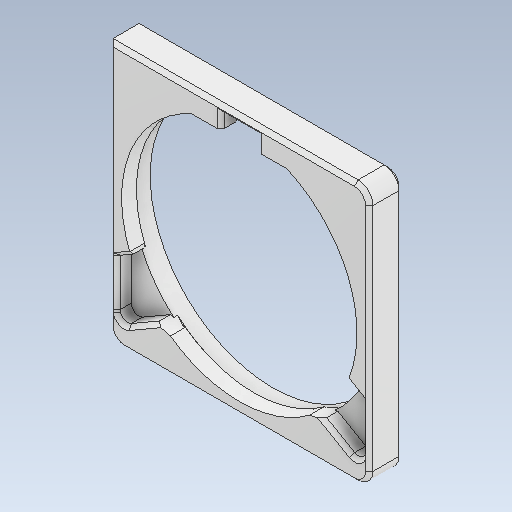
# Autodesk Inventor part: DD3_Zentrierhilfe
Saved by Autodesk Inventor 2020.2 (Build 242310000, 310)
## iProperties
Created: 2021-09-17
Part Number: DD3_Zentrierhilfe
Material: PC/ABS-Kunststoff
Document SubType Name: Modeling
Designer: johan
Density: 0.357273 g/cm^3
Appearance: Glatt - Weiß
Author: johan
Autodesk Inventor part; units mm, degrees
ref_plane "YZ Plane" through (0, 0, 0) normal (1, 0, 0) x (0, 1, 0)
ref_plane "XZ Plane" through (0, 0, 0) normal (0, 1, 0) x (-1, 0, 0)
sketch "Skizze1" plane through (0, 0, 0) normal (0, 0, 1) x (1, 0, 0)
  line L0 (-17, 17) -> (15.5, 17) construction
  line L1 (-17, -15.5) -> (-17, 17) construction
  arc A0 (-17, -15.5) -> (-15.5, -17) centre (-15.5, -15.5) ccw construction
  line L2 (15.5, -17) -> (-15.5, -17) construction
  arc A1 (15.5, -17) -> (17, -15.5) centre (15.5, -15.5) ccw construction
  line L3 (17, 15.5) -> (17, -15.5) construction
  arc A2 (17, 15.5) -> (15.5, 17) centre (15.5, 15.5) ccw construction
  arc A3 (-6.48479, 14.9) -> (6.48479, 14.9) centre (0, 0) ccw
  line L4 (6.48479, 14.9) -> (-6.48479, 14.9)
  line L5 (-2.5, 16.9) -> (2.5, 16.9)
  line L6 (2.5, 16.9) -> (2.5, 14.9)
  line L7 (2.5, 14.9) -> (-2.5, 14.9)
  line L8 (-2.5, 14.9) -> (-2.5, 16.9)
  line L9 (0, 0) -> (0, 20.018159) construction
  line L10 (0, 0) -> (0, -16.25) construction
  line L11 (0, 0) -> (-16.25, 0) construction
  line L12 (0, 0) -> (16.25, 0) construction
  line L13 (-16.5, -7.283583) -> (-13, -13.345761)
  line L14 (-13, -13.345761) -> (-11.267949, -12.345761)
  line L15 (-11.267949, -12.345761) -> (-14.767949, -6.283583)
  line L16 (-14.767949, -6.283583) -> (-16.5, -7.283583)
  line L17 (16.5, -7.283583) -> (13, -13.345761)
  line L18 (13, -13.345761) -> (11.267949, -12.345761)
  line L19 (11.267949, -12.345761) -> (14.767949, -6.283583)
  line L20 (14.767949, -6.283583) -> (16.5, -7.283583)
  line L21 (15.5, 17.5) -> (-17.5, 17.5)
  arc A4 (17.5, 15.5) -> (15.5, 17.5) centre (15.5, 15.5) ccw
  line L22 (17.5, -15.5) -> (17.5, 15.5)
  arc A5 (15.5, -17.5) -> (17.5, -15.5) centre (15.5, -15.5) ccw
  line L23 (-15.5, -17.5) -> (15.5, -17.5)
  arc A6 (-17.5, -15.5) -> (-15.5, -17.5) centre (-15.5, -15.5) ccw
  line L24 (-17.5, 17.5) -> (-17.5, -15.5)
  arc A7 (-6.400976, 14.5) -> (6.400976, 14.5) centre (0, 0) ccw
  line L25 (-6.400976, 14.5) -> (6.400976, 14.5)
  line L26 (-2.5, 14.9) -> (-2.5, 14.5)
  line L27 (2.5, 14.9) -> (2.5, 14.5)
  line L28 (14.767949, -6.283583) -> (14.767949, -5.755882)
  line L29 (11.267949, -12.345761) -> (9.430948, -12.738906)
  line L30 (-11.267949, -12.345761) -> (-9.284876, -12.845761)
  line L31 (-14.767949, -6.283583) -> (-14.767949, -5.755882)
  line L32 (13, -13.345761) -> (15.047939, -14.528139)
  line L33 (16.547911, -13.654594) -> (16.5, -7.283583)
  arc A8 (15.047939, -14.528139) -> (16.547911, -13.654594) centre (15.547939, -13.662114) ccw
  line L34 (-13, -13.345761) -> (-15.047939, -14.528139)
  line L35 (-16.547911, -13.654594) -> (-16.5, -7.283583)
  arc A9 (-16.547911, -13.654594) -> (-15.047939, -14.528139) centre (-15.547939, -13.662114) ccw
  point P0 (0, 0)
  point P1 (14.943148, -6.384734)
  point P2 (12.195347, -10.73946)
  point P3 (-12.195347, -10.73946)
  point P4 (-14.943148, -6.384734)
  dimension "d0" = 5
  dimension "d1" = 2
  dimension "d2" = 7
  dimension "d4" = 2
  dimension "d5" = 60
  dimension "d6" = 16.5
  dimension "d8" = 14.9
  dimension "d16" = 0.4
  dimension "d17" = 102.08
  dimension "d18" = 75.8487
  dimension "d19" = 20.23116
  dimension "d20" = 2.55685
  dimension "d21" = 23.88473
  dimension "d22" = 5.30465
  dimension "d23" = 28.23946
  dimension "d24" = 15
  dimension "d25" = 2.6
  dimension "d26" = 2.51816
  dimension "d27" = 20
  dimension "d28" = 2.6
  dimension "d29" = 29.69535
  dimension "d30" = 28.23946
  dimension "d31" = 32.44315
  dimension "d32" = 23.88473
  dimension "d36" = 1
  dimension "d37" = 0.43087
  constraints: 54 end point, 13 point on circle, 7 symmetric about line, 5 parallel, 5 perpendicular, 3 centre point, 3 point on line, 3 tangent, 2 vertical, 1 horizontal, 3 other
  measures "d0" distance of L6.end L7.end
  measures "d1" distance of L5.end L6.end
  measures "d2" distance of L13.start L13.end
  measures "d4" distance of L14.end L13.end
  measures "d5" angle of L13 L5
  measures "d6" distance from line of L10 L13.start
  measures "d8" distance from line of L7 point (0, 0)
  measures "d16" radial gap between concentric circles of A3 A7
  measures "d17" angle of L22 L29
  measures "d18" angle of L22 L30
  measures "d19" distance from line of L22.end L20
  measures "d20" distance from line of point (14.943, -6.385) L22
  measures "d21" distance from line of point (14.943, -6.385) L21
  measures "d22" distance from line of point (12.195, -10.739) L22
  measures "d23" distance from line of point (12.195, -10.739) L21
  measures "d24" distance from line of point (2.5, 14.9) L22
  measures "d25" distance from line of point (2.5, 14.9) L21
  measures "d26" distance from line of L9.end L21
  measures "d27" distance from line of point (-2.5, 14.9) L22
  measures "d28" distance from line of point (-2.5, 14.9) L21
  measures "d29" distance from line of point (-12.195, -10.739) L22
  measures "d30" distance from line of point (-12.195, -10.739) L21
  measures "d31" distance from line of point (-14.943, -6.385) L22
  measures "d32" distance from line of point (-14.943, -6.385) L21
  measures "d36" radius of A8
  measures "d37" angle of L3 L33
extrude "Extrusion1" add sketch "Skizze1" against normal blind 2 contours L4 L26 L25 A7 L31 L16 A3 | L4 A3 L20 L28 A7 L25 L27 | L30 A7 L29 A3 | A4 L22 A5 L23 A6 L24 L21
sketch "Skizze2" plane through (0, 0, -2) normal (0, 0, -1) x (-1, 0, 0)
  arc A0 (-15.5, 17.5) -> (-17.5, 15.5) centre (-15.5, 15.5) ccw
  line L0 (17.5, 17.5) -> (-15.5, 17.5)
  line L1 (17.5, -15.5) -> (17.5, 17.5)
  arc A1 (15.5, -17.5) -> (17.5, -15.5) centre (15.5, -15.5) ccw
  line L2 (-15.5, -17.5) -> (15.5, -17.5)
  arc A2 (-17.5, -15.5) -> (-15.5, -17.5) centre (-15.5, -15.5) ccw
  line L3 (-17.5, 15.5) -> (-17.5, -15.5)
  line L4 (-16.68909, 13.34859) -> (-15.622361, 15.139421)
  arc A3 (-15.192794, 15.139421) -> (-15.622361, 15.139421) centre (-15.407577, 15.011483) ccw
  line L5 (-15.192794, 15.139421) -> (-14.126064, 13.34859)
  arc A4 (-14.340848, 12.970652) -> (-14.126064, 13.34859) centre (-14.340848, 13.220652) ccw
  line L6 (-14.340848, 12.970652) -> (-14.557577, 12.970652)
  arc A5 (-14.557577, 12.970652) -> (-14.807577, 12.720652) centre (-14.557577, 12.720652) ccw
  line L7 (-14.807577, 12.720652) -> (-14.807577, 9.779497)
  arc A6 (-15.057577, 9.529497) -> (-14.807577, 9.779497) centre (-15.057577, 9.779497) ccw
  line L8 (-15.057577, 9.529497) -> (-15.757577, 9.529497)
  arc A7 (-16.68909, 13.34859) -> (-16.474307, 12.970652) centre (-16.474307, 13.220652) ccw
  line L9 (-16.257577, 12.970652) -> (-16.474307, 12.970652)
  arc A8 (-16.007577, 12.720652) -> (-16.257577, 12.970652) centre (-16.257577, 12.720652) ccw
  line L10 (-16.007577, 9.779497) -> (-16.007577, 12.720652)
  arc A9 (-16.007577, 9.779497) -> (-15.757577, 9.529497) centre (-15.757577, 9.779497) ccw
  line L11 (-15.057577, 9.529497) -> (-15.757577, 9.529497)
  arc A10 (-15.057577, 9.529497) -> (-14.807577, 9.779497) centre (-15.057577, 9.779497) ccw
  line L12 (-14.807577, 12.720652) -> (-14.807577, 9.779497)
  arc A11 (-14.557577, 12.970652) -> (-14.807577, 12.720652) centre (-14.557577, 12.720652) ccw
  line L13 (-14.340848, 12.970652) -> (-14.557577, 12.970652)
  arc A12 (-14.340848, 12.970652) -> (-14.126064, 13.34859) centre (-14.340848, 13.220652) ccw
  line L14 (-15.192794, 15.139421) -> (-14.126064, 13.34859)
  arc A13 (-15.192794, 15.139421) -> (-15.622361, 15.139421) centre (-15.407577, 15.011483) ccw
  line L15 (-16.68909, 13.34859) -> (-15.622361, 15.139421)
  line L16 (-15.5, 17) -> (17, 17)
  arc A14 (-15.5, 17) -> (-17, 15.5) centre (-15.5, 15.5) ccw
  line L17 (-17, -15.5) -> (-17, 15.5)
  arc A15 (-17, -15.5) -> (-15.5, -17) centre (-15.5, -15.5) ccw
  line L18 (15.5, -17) -> (-15.5, -17)
  arc A16 (15.5, -17) -> (17, -15.5) centre (15.5, -15.5) ccw
  line L19 (17, 17) -> (17, -15.5)
  arc A17 (-14.557577, 12.970652) -> (-14.807577, 12.720652) centre (-14.557577, 12.720652) ccw
  line L20 (-14.807577, 12.720652) -> (-14.807577, 9.779497)
  arc A18 (-15.057577, 9.529497) -> (-14.807577, 9.779497) centre (-15.057577, 9.779497) ccw
  line L21 (-15.057577, 9.529497) -> (-15.757577, 9.529497)
  arc A19 (-16.007577, 9.779497) -> (-15.757577, 9.529497) centre (-15.757577, 9.779497) ccw
  line L22 (-16.007577, 9.779497) -> (-16.007577, 12.720652)
  arc A20 (-16.007577, 12.720652) -> (-16.257577, 12.970652) centre (-16.257577, 12.720652) ccw
  line L23 (-16.257577, 12.970652) -> (-16.474307, 12.970652)
  arc A21 (-16.68909, 13.34859) -> (-16.474307, 12.970652) centre (-16.474307, 13.220652) ccw
  line L24 (-16.68909, 13.34859) -> (-15.622361, 15.139421)
  arc A22 (-15.192794, 15.139421) -> (-15.622361, 15.139421) centre (-15.407577, 15.011483) ccw
  line L25 (-15.192794, 15.139421) -> (-14.126064, 13.34859)
  arc A23 (-14.340848, 12.970652) -> (-14.126064, 13.34859) centre (-14.340848, 13.220652) ccw
  line L26 (-14.340848, 12.970652) -> (-14.557577, 12.970652)
  line L27 (7.088018, 14.9) -> (-7.088018, 14.9)
  arc A24 (-7.088018, 14.9) -> (7.088018, 14.9) centre (0, 0) ccw
  point P0 (0, 0)
ref_plane "Arbeitsebene1" through (-17, -17, -4.5) normal (0, 0, -1) x (0, 1, 0)
extrude "Extrusion2" add sketch "Skizze2" along normal up to surface (2.5 mm away) contours L0 L1 A1 L2 A2 L3 A0 | L16 L19 A16 L18 A15 L17 A14
chamfer "Fase1" distance 0.5 angle 45 20 edges at (-1, 17.5, -4.5) (16.9142, 16.9142, -4.5) (17.5, 0, -4.5) (16.9142, -16.9142, -4.5) (0, -17.5, -4.5) (-16.9142, -16.9142, -4.5) (-17.5, 1, -4.5) (-17.5, 1, 0) (-16.9142, -16.9142, 0) (0, -17.5, 0) (16.9142, -16.9142, 0) (17.5, 0, 0) (16.9142, 16.9142, 0) (-1, 17.5, 0) (15.634, -6.7836, 0) (13.1579, -13.4369, 0) (-13.1579, -13.4369, 0) (-15.634, -6.7836, 0) (2.5, 15.7, 0) (-2.5, 15.7, 0)
chamfer "Fase2" distance 0.5 angle 45 5 edges at (15.4389, 5.8215, -2) (-15.4389, 5.8215, -2) (0.0174, -16.5, -2) (4.794, 14.9, -2) (-4.794, 14.9, -2)
